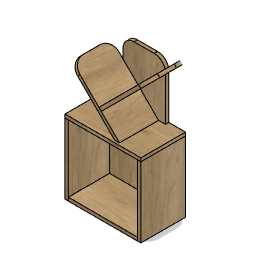
Project 02 (Autodesk Fusion 360 design; units mm, degrees)
Autodesk Fusion 360 part; units mm, degrees
note: some values were not read from the file. Set by a fixed rule: which sketch regions a step uses.
sketch "Sketch1" plane through (0, 0, 0) normal (0, 1, 0) x (1, 0, 0)
  line L0 (0, 0) -> (340, 0)
  line L1 (340, 0) -> (340, -200)
  line L2 (340, -200) -> (0, -200)
  line L3 (0, -200) -> (0, 0)
  line L4 (0, 0) -> (15, 0)
  line L5 (15, 0) -> (15, -200)
  line L6 (15, -200) -> (0, -200)
  line L7 (0, -200) -> (0, 0)
  line L8 (340, 0) -> (325, 0)
  line L9 (325, 0) -> (325, -200)
  line L10 (325, -200) -> (340, -200)
  line L11 (340, -200) -> (340, 0)
  line L12 (15, 0) -> (325, 0)
  line L13 (325, 0) -> (325, -15)
  line L14 (325, -15) -> (15, -15)
  line L15 (15, -15) -> (15, 0)
  dimension "d1" = 340
  dimension "d2" = 200
  dimension "d3" = 15
  dimension "d4" = 15
  dimension "d5" = 15
  constraint horizontal L0
  constraint vertical L1
  constraint horizontal L2
  constraint vertical L3
  constraint coincident L0.start L3.end
  constraint horizontal L4
  constraint vertical L5
  constraint horizontal L6
  constraint vertical L7
  constraint coincident L2 L5.end
  constraint horizontal L8
  constraint vertical L9
  constraint horizontal L10
  constraint vertical L11
  constraint coincident L2 L9.end
  constraint horizontal L12
  constraint vertical L13
  constraint horizontal L14
  constraint vertical L15
  constraint coincident L9 L13.end
  measures "d1" distance of L0.start L0.end
  measures "d2" distance of L0.start L2.end
  measures "d3" distance of L0.start L4.end
  measures "d4" distance of L0.end L8.end
  measures "d5" distance of L4.end L14.end
extrude "Extrude1" add sketch "Sketch1" along normal blind 540 contours L0 L5 L9 L12 L13 L14 L15 makes body 1
extrude "Extrude2" add sketch "Sketch1" along normal blind 540 separate body contours L0 L2 L3 L4 L5 L6 L7 L15 makes body 2
extrude "Extrude3" add sketch "Sketch1" along normal blind 540 separate body contours L0 L1 L2 L8 L9 L10 L11 L13 makes body 3
sketch "Sketch2" plane through (15, 0, 0) normal (1, 0, 0) x (0, 0, -1)
  line L0 (-200, 0) -> (0, 0)
  line L1 (0, 0) -> (0, 540)
  line L2 (0, 540) -> (-200, 540)
  line L3 (-200, 540) -> (-200, 0)
  line L4 (-15, 225) -> (-200, 225)
  line L5 (-200, 225) -> (-200, 240)
  line L6 (-200, 240) -> (-15, 240)
  line L7 (-15, 240) -> (-15, 225)
  dimension "d14" = 15
  constraint horizontal L4
  constraint vertical L5
  constraint horizontal L6
  constraint vertical L7
  constraint coincident L3 L5.end
  measures "d14" distance of L4.start L6.end
extrude "Extrude5" add sketch "Sketch2" along normal blind 310 separate body contours L3 L4 L5 L6 L7 makes body 4
sketch "Sketch3" plane through (0, 540, 0) normal (0, 1, 0) x (-1, 0, 0)
  line L0 (-15, 200) -> (-15, 0)
  line L1 (-15, 0) -> (0, 0)
  line L2 (0, 0) -> (0, 200)
  line L3 (0, 200) -> (-15, 200)
  line L4 (0, 0) -> (-340, 0)
  line L5 (-340, 0) -> (-340, 200)
  line L6 (-340, 200) -> (0, 200)
  line L7 (0, 200) -> (0, 0)
  constraint horizontal L4
  constraint vertical L5
  constraint horizontal L6
  constraint vertical L7
  constraint coincident L1.end L2.start
extrude "Extrude6" add sketch "Sketch3" along normal blind 15 separate body makes body 5
sketch "Sketch4" plane through (0, 555, 0) normal (0, 1, 0) x (-1, 0, 0)
  line L0 (0, 200) -> (-340, 200)
  line L1 (-340, 200) -> (-340, 0)
  line L2 (-340, 0) -> (0, 0)
  line L3 (0, 0) -> (0, 200)
  line L4 (-75, 0) -> (-265, 0)
  line L5 (-265, 0) -> (-265, 15)
  line L6 (-265, 15) -> (-75, 15)
  line L7 (-75, 15) -> (-75, 0)
  dimension "d19" = 15
  constraint horizontal L4
  constraint vertical L5
  constraint horizontal L6
  constraint vertical L7
  constraint coincident L2 L4.start
  measures "d19" distance of L4.start L6.end
extrude "Extrude7" add sketch "Sketch4" along normal blind 250 separate body contours L2 L4 L5 L6 L7 makes body 6
sketch "Sketch5" plane through (0, 0, 15) normal (0, 0, 1) x (1, 0, 0)
  line L0 (75, 555) -> (265, 555)
  line L1 (265, 555) -> (265, 805)
  line L2 (265, 805) -> (75, 805)
  line L3 (75, 805) -> (75, 555)
  line L4 (0, 555) -> (170, 555) construction
  line L5 (170, 555) -> (234, 555) construction
  line L6 (234, 555) -> (21.868, 767.132)
  line L7 (234, 555) -> (494, 555) construction
  line L8 (21.868, 767.132) -> (11.2614, 756.5254)
  line L9 (11.2614, 756.5254) -> (212.7868, 555)
  line L10 (11.2614, 756.5254) -> (284.5456, 756.5254) construction
  line L11 (234, 555) -> (152.6827, 636.3173) construction
  line L12 (152.6827, 636.3173) -> (364.8148, 848.4493)
  line L13 (364.8148, 848.4493) -> (354.2082, 859.0559)
  line L14 (354.2082, 859.0559) -> (142.0761, 646.9239)
  dimension "d22" = 64
  dimension "d23" = 135
  dimension "d24" = 300
  dimension "d25" = 15
  dimension "d26" = 45
  dimension "d27" = 115
  dimension "d28" = 90
  dimension "d29" = 300
  dimension "d30" = 15
  constraint midpoint L0 L4.end
  constraint parallel L0 L4
  constraint coincident L0 L5.end
  constraint horizontal L7
  constraint perpendicular L6 L8
  constraint horizontal L10
  constraint coincident L5 L9.end
  constraint coincident L6 L11.end
  constraint perpendicular L12 L13
  constraint coincident L6 L14.end
  constraint perpendicular L6 L14
  measures "d22" distance of L4.end L5.end
  measures "d23" angle of L6 L7
  measures "d24" distance of L5.end L6.end
  measures "d25" distance of L6.end L8.end
  measures "d26" angle of L9 L10
  measures "d27" distance of L5.end L11.end
  measures "d28" angle of L11 L12
  measures "d29" distance of L11.end L12.end
  measures "d30" distance of L12.end L13.end
extrude "Extrude8" add sketch "Sketch5" along normal blind 175 separate body contours L0 L3 L6 L9 | L3 L6 L8 L9 makes body 7
extrude "Extrude9" add sketch "Sketch5" along normal blind 175 separate body contours L1 L6 L12 L14 | L1 L12 L13 L14 makes body 8
fillet "Fillet1" radius 50 2 edges at (265, 805, 7.5) (75, 805, 7.5) on bodies 6
fillet "Fillet2" radius 50 4 edges at (16.5647, 761.8287, 190) (16.5647, 761.8287, 15) (359.5115, 853.7526, 190) (359.5115, 853.7526, 15) on bodies 7 8
extrude "Extrude10" add 2 faces at (5, 0, 71.6667) (335, 0, 71.6667) along direction (0, -1, 0) blind 90 on bodies 2 3 bodies 2 3 4 5 6 7 8
extrude "Extrude11" add 1 faces at (118.3333, 0, 5) along direction (0, -1, 0) blind 90 on bodies 1 bodies 1
move_body "Move1" bodies 2 3 7 4 5 6 8 1 to x (1, 0, 0) y (0, 1, 0) z (0, 0, 1) at (0, 90, 0)
extrude "Extrude13" cut 1 faces at (118.3333, 0, 5) along direction (0, 1, 0) blind 315 on bodies 1 bodies 1
extrude "Extrude14" cut 1 faces at (5, 0, 66.6667) along direction (0, 1, 0) blind 315 on bodies 2 bodies 2
extrude "Extrude15" cut 1 faces at (330, 0, 66.6667) along direction (0, 1, 0) blind 315 on bodies 3 bodies 3
move_body "Move2" bodies 1 2 5 8 7 6 3 4 to x (1, 0, 0) y (0, 1, 0) z (0, 0, 1) at (0, -315, 0)
